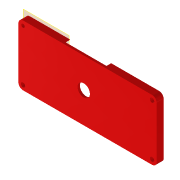
# Autodesk Inventor part: ESP32ParasiteMicroscope_top_v0
Saved by Autodesk Inventor 2022 (Build 260153000, 153)
## iProperties
Created: 2022-02-02
Part Number: ESP32ParasiteMicroscope_top_v0
Material: Generisch
Document SubType Name: Modeling
Designer: diederichbenedict
Density: 1 g/cm^3
Appearance: Rot
Author: diederichbenedict
Autodesk Inventor part; units mm, degrees
ref_plane "YZ Plane" through (0, 0, 0) normal (1, 0, 0) x (0, 1, 0)
ref_plane "XZ Plane" through (0, 0, 0) normal (0, 1, 0) x (-1, 0, 0)
ref_plane "XY Plane" through (0, 0, 0) normal (0, 0, 1) x (1, 0, 0)
ref_plane "Arbeitsebene1" through (0, 0, 0) normal (0, 0, 1) x (1, 0, 0)
sketch "Skizze1" plane through (0, 0, 0) normal (0, 0, 1) x (1, 0, 0)
  line L0 (-19.6031, 19.4874) -> (14.7153, 19.4874)
  line L1 (14.7153, -19.4874) -> (-19.6031, -19.4874)
  spline S0 degree 3 poles (15.9885, -12.7941) (15.1267, -14.0688) (14.121, -15.2558) (11.7288, -17.5435) (10.3143, -18.6047) (8.791, -19.4874) knots 0 0 0 0 0.461588 0.461588 0.987001 0.987001 0.987001 0.987001 projected
  line L2 (8.791, -19.4874) -> (41.5374, -19.4874) projected
  arc A0 (41.5374, -19.4874) -> (44.5374, -16.4874) centre (41.5374, -16.4874) ccw projected
  line L3 (44.5374, -16.4874) -> (44.5374, 16.4874) projected
  arc A1 (44.5374, 16.4874) -> (41.5374, 19.4874) centre (41.5374, 16.4874) ccw projected
  line L4 (41.5374, 19.4874) -> (7.7659, 19.4874) projected
  arc A2 (9.8338, 18.2553) -> (7.7659, 19.4874) centre (-2.4439, 0) ccw projected
  spline S1 degree 3 poles (9.8338, 18.2553) (12.0089, 16.8318) (13.9164, 15.0326) (17.1857, 10.6246) (18.4338, 7.9941) (19.8573, 2.3897) (20.014, -0.5318) (19.3704, -5.0763) (18.9435, -6.7188) (17.7261, -9.8803) (16.9385, -11.3888) (15.9885, -12.7941) knots 0.079909 0.079909 0.079909 0.079909 0.861026 0.861026 1.726159 1.726159 2.595399 2.595399 3.102699 3.102699 3.611409 3.611409 3.611409 3.611409 projected
  circle A3 centre (41.5374, 16.4874) radius 1.4 projected
  circle A4 centre (41.5374, -16.4874) radius 1.4 projected
  line L5 (7.9526, -13.3626) -> (-30.0474, -13.3626) projected
  spline S2 degree 3 poles (-21.9975, -11.0045) (-23.3957, -8.4471) (-24.2821, -5.6417) (-24.9256, 0.1377) (-24.6818, 3.0555) (-23.0907, 8.6196) (-21.7637, 11.2138) (-18.9405, 14.7925) (-17.7594, 15.9834) (-15.3624, 17.9058) (-14.189, 18.6758) (-12.951, 19.3288) knots 0 0 0 0 0.874402 0.874402 1.744697 1.744697 2.610882 2.610882 3.112603 3.112603 3.533005 3.533005 3.533005 3.533005 projected
  arc A5 (-12.6537, 19.4874) -> (-12.951, 19.3288) centre (-2.4439, 0) ccw projected
  line L6 (-12.6537, 19.4874) -> (-41.5374, 19.4874) projected
  arc A6 (-41.5374, 19.4874) -> (-44.5374, 16.4874) centre (-41.5374, 16.4874) ccw projected
  line L7 (-44.5374, 16.4874) -> (-44.5374, -16.4874) projected
  arc A7 (-44.5374, -16.4874) -> (-41.5374, -19.4874) centre (-41.5374, -16.4874) ccw projected
  line L8 (-41.5374, -19.4874) -> (-13.6864, -19.4874) projected
  spline S3 degree 3 poles (-13.6864, -19.4874) (-15.5675, -18.3989) (-17.2815, -17.0397) (-20.0302, -14.1081) (-21.1203, -12.6091) (-21.9975, -11.0045) knots 0.10415 0.10415 0.10415 0.10415 0.757219 0.757219 1.31027 1.31027 1.31027 1.31027 projected
  circle A8 centre (-41.5374, -16.4874) radius 1.4 projected
  circle A9 centre (-41.5374, 16.4874) radius 1.15 projected
  spline S4 degree 3 poles (-24.8057, 2.4903) (-24.4907, 5.3187) (-23.6418, 8.0626) (-20.9263, 13.1619) (-19.0572, 15.4543) (-14.5454, 19.1935) (-11.9459, 20.6045) (-6.3523, 22.3508) (-3.4117, 22.6693) (2.426, 22.1612) (5.2673, 21.3394) (10.4751, 18.653) (12.7917, 16.814) (16.5896, 12.3516) (18.0345, 9.7708) (19.8538, 4.2005) (20.2108, 1.2643) (19.7791, -4.5795) (18.9946, -7.4314) (16.3765, -12.6738) (14.568, -15.0143) (10.1556, -18.8702) (7.5939, -20.3489) (2.048, -22.2409) (-0.8833, -22.6362) (-6.7323, -22.281) (-9.5942, -21.5339) (-14.8704, -18.9846) (-17.2344, -17.2069) (-21.1477, -12.8453) (-22.6597, -10.3032) (-24.6241, -4.7825) (-25.0578, -1.8567) (-24.7791, 3.9965) (-24.0695, 6.8679) (-21.5895, 12.1771) (-19.8428, 14.564) (-15.5329, 18.5341) (-13.0107, 20.0793) (-7.5162, 22.1157) (-4.5963, 22.5876) (1.26, 22.3856) (4.1405, 21.7136) (9.4816, 19.3033) (11.8912, 17.588) (15.9174, 13.3303) (17.4954, 10.8286) (19.6036, 5.3612) (20.1136, 2.4477) (19.9882, -3.4108) (19.354, -6.2997) (17.0137, -11.672) (15.3301, -14.1038) (11.1255, -18.1853) (8.6447, -19.7959) (3.2053, -21.9755) (0.2987, -22.5236) (-5.5609, -22.4748) (-8.4579, -21.8784) (-13.8603, -19.6087) (-16.314, -17.957) (-20.4501, -13.8062) (-22.093, -11.3466) (-24.3436, -5.9362) (-24.9297, -3.0371) (-24.9576, 2.8227) (-24.3992, 5.7272) (-22.2003, 11.1588) (-20.5809, 13.6339) (-16.4845, 17.824) (-14.0467, 19.499) (-8.6662, 21.8201) (-5.7749, 22.4441) (0.0839, 22.5487) (2.9956, 22.0283) (8.4555, 19.9007) (10.9516, 18.3138) (15.1949, 14.2726) (16.9016, 11.8569) (19.2929, 6.5072) (19.9547, 3.6244) (20.1359, -2.2326) (19.6537, -5.1508) (17.5977, -10.6381) (16.0436, -13.1547) (12.0582, -17.4506) (9.665, -19.1887) (4.3471, -21.6499) (1.4732, -22.3493) (-4.3809, -22.6071) (-7.3052, -22.1631) (-12.8189, -20.1791) (-15.3556, -18.658) (-19.7032, -14.7292) (-21.4726, -12.359) (-24.0031, -7.0737) (-24.74, -4.2092) (-25.0745, 1.6411) (-24.6687, 4.5709) (-22.757, 10.1101) (-21.2693, 12.6665) (-17.3977, 17.0651) (-15.0508, 18.8653) (-9.7991, 21.4648) (-6.9445, 22.2391) (-1.0991, 22.6501) (1.8358, 22.2827) (7.3995, 20.4436) (9.9752, 18.9895) (14.4241, 15.1758) (16.2549, 12.8526) (18.9228, 7.6354) (19.7344, 4.7911) (20.2218, -1.0484) (19.8929, -3.9878) (18.1267, -9.5751) (16.7064, -12.1696) (12.9512, -16.668) (10.6523, -18.529) (6.0021, -20.9842) (3.7866, -21.7452) (-0.7988, -22.5603) (-3.1408, -22.6094) (-5.4486, -22.2985) knots 17.60465 17.60465 17.60465 17.60465 18.45888 18.45888 19.337874 19.337874 20.216868 20.216868 21.095862 21.095862 21.974857 21.974857 22.853851 22.853851 23.732845 23.732845 24.61184 24.61184 25.490834 25.490834 26.369828 26.369828 27.248822 27.248822 28.127817 28.127817 29.006811 29.006811 29.885805 29.885805 30.764799 30.764799 31.643794 31.643794 32.522788 32.522788 33.401782 33.401782 34.280777 34.280777 35.159771 35.159771 36.038765 36.038765 36.917759 36.917759 37.796754 37.796754 38.675748 38.675748 39.554742 39.554742 40.433736 40.433736 41.312731 41.312731 42.191725 42.191725 43.070719 43.070719 43.949713 43.949713 44.828708 44.828708 45.707702 45.707702 46.586696 46.586696 47.465691 47.465691 48.344685 48.344685 49.223679 49.223679 50.102673 50.102673 50.981668 50.981668 51.860662 51.860662 52.739656 52.739656 53.61865 53.61865 54.497645 54.497645 55.376639 55.376639 56.255633 56.255633 57.134628 57.134628 58.013622 58.013622 58.892616 58.892616 59.77161 59.77161 60.650605 60.650605 61.529599 61.529599 62.408593 62.408593 63.287587 63.287587 64.166582 64.166582 65.045576 65.045576 65.92457 65.92457 66.803564 66.803564 67.682559 67.682559 68.561553 68.561553 69.440547 69.440547 70.139143 70.139143 70.83774 70.83774 70.83774 70.83774 projected
  point P0 (0, 0)
  constraints: 4 end point, 1 horizontal, 1 parallel
extrude "Extrusion1" add sketch "Skizze1" along normal blind 4.5 contours A5 S2 S3 L5 S4 L0 | L0 A2 S1 S0 L1 S3 S2 A5 | L0 S4 L1 S0 S1 A2 | S4 L1 L8 A7 L7 A6 L6 L0 | L0 L4 A1 L3 A0 L2 L1 S4 | L5 S3 S4
sketch "Skizze2" plane through (0, 0, 0) normal (0, 0, -1) x (-1, 0, 0)
  spline S0 degree 3 poles (-8.6773, -19.4874) (-12.6741, -17.2065) (-15.9385, -13.664) (-17.8858, -9.4945) (-19.8263, -5.3394) (-20.4501, -0.581) (-19.646, 3.9338) (-18.841, 8.4547) (-16.6079, 12.7105) (-13.3453, 15.9419) (-11.953, 17.3208) (-10.3792, 18.5162) (-8.6773, 19.4874) knots 3.660178 3.660178 3.660178 3.660178 4.275468 4.275468 4.275468 4.888623 4.888623 4.888623 5.502599 5.502599 5.502599 5.7646 5.7646 5.7646 5.7646 projected
  spline S1 degree 3 poles (15.6702, -17.7105) (12.0344, -20.4258) (7.5456, -21.981) (3.0092, -22.097) (-1.5262, -22.2131) (-6.0878, -20.89) (-9.8573, -18.3651) (-13.6261, -15.8408) (-16.5853, -12.127) (-18.2044, -7.8897) (-19.8231, -3.6532) (-20.0946, 1.0867) (-18.9702, 5.4804) (-17.846, 9.8732) (-15.3316, 13.8993) (-11.8776, 16.8372) (-8.4243, 19.7746) (-4.0479, 21.6104) (0.4676, 22.0157) (4.9823, 22.421) (9.6148, 21.3945) (13.5357, 19.1199) (17.4559, 16.8457) (20.6463, 13.3346) (22.5357, 9.2152) (24.4248, 5.0964) (25.0045, 0.3887) (24.1711, -4.0654) (23.3017, -8.7119) (20.8952, -13.0574) (17.4179, -16.2597) (14.0494, -19.3619) (9.6951, -21.3773) (5.1502, -21.938) (0.6241, -22.4963) (-4.0691, -21.6096) (-8.0795, -19.4385) (-12.0876, -17.2687) (-15.3943, -13.8264) (-17.4015, -9.7344) (-19.4075, -5.6447) (-20.1058, -0.9257) (-19.3702, 3.5696) (-18.635, 8.0626) (-16.4709, 12.3107) (-13.2688, 15.547) (-10.0683, 18.7816) (-5.8461, 20.99) (-1.3638, 21.7738) (3.1163, 22.5573) (7.8349, 21.9139) (11.9417, 19.9597) (16.0466, 18.0064) (19.5207, 14.7528) (21.7387, 10.7848) (23.9556, 6.8185) (24.907, 2.1572) (24.4218, -2.3606) (23.9368, -6.8763) (22.0187, -11.2274) (19.0123, -14.6317) (16.0072, -18.0346) (11.9289, -20.4754) (7.5099, -21.5159) (3.0927, -22.556) (-1.6441, -22.1919) (-5.8505, -20.4891) (-10.0553, -18.7869) (-13.7102, -15.755) (-16.16, -11.9371) (-18.6088, -8.1206) (-19.8418, -3.5366) (-19.638, 0.9934) (-19.4343, 5.5218) (-17.7958, 9.975) (-15.0159, 13.5556) (-12.2369, 17.1349) (-8.3304, 19.8254) (-3.9954, 21.1455) (0.4165, 22.4891) (5.2511, 22.4051) (9.6138, 20.9091) (13.9256, 19.4306) (17.7557, 16.5809) (20.4109, 12.8758) (23.0632, 9.1748) (24.5305, 4.6381) (24.548, 0.0849) (24.5655, -4.4636) (23.136, -9.0069) (20.5173, -12.726) (17.9011, -16.4415) (14.1104, -19.3169) (9.8272, -20.8347) (5.5477, -22.3513) (0.7969, -22.5055) (-3.572, -21.2699) (-7.9373, -20.0352) (-11.9008, -17.4187) (-14.7514, -13.8896) (-17.6, -10.363) (-19.3241, -5.9418) (-19.6148, -1.4178) (-19.9144, 3.2433) (-18.6883, 7.9901) (-16.1689, 11.9231) (-13.7125, 15.7579) (-10.0405, 18.801) (-5.8164, 20.5028) (-1.6007, 22.2013) (3.1447, 22.5558) (7.5659, 21.5026) (11.9796, 20.4513) (16.0494, 18.0021) (19.0451, 14.5945) (22.1911, 11.016) (24.1323, 6.3965) (24.4869, 1.6449) (24.8252, -2.8882) (23.7216, -7.5182) (21.3749, -11.4113) (19.0355, -15.2922) (15.4721, -18.4228) (11.3223, -20.2429) (7.1708, -22.0637) (2.452, -22.5643) (-1.9891, -21.6552) (-2.6592, -21.518) (-3.3229, -21.3497) (-3.9774, -21.151) knots 24.602078 24.602078 24.602078 24.602078 25.217953 25.217953 25.217953 25.833709 25.833709 25.833709 26.449348 26.449348 26.449348 27.064873 27.064873 27.064873 27.680287 27.680287 27.680287 28.295593 28.295593 28.295593 28.910794 28.910794 28.910794 29.525892 29.525892 29.525892 30.140891 30.140891 30.140891 30.782458 30.782458 30.782458 31.403975 31.403975 31.403975 32.022909 32.022909 32.022909 32.641484 32.641484 32.641484 33.259714 33.259714 33.259714 33.87761 33.87761 33.87761 34.495185 34.495185 34.495185 35.11245 35.11245 35.11245 35.729418 35.729418 35.729418 36.346101 36.346101 36.346101 36.962511 36.962511 36.962511 37.578659 37.578659 37.578659 38.194557 38.194557 38.194557 38.810218 38.810218 38.810218 39.425653 39.425653 39.425653 40.040873 40.040873 40.040873 40.65589 40.65589 40.65589 41.281836 41.281836 41.281836 41.900486 41.900486 41.900486 42.518451 42.518451 42.518451 43.13578 43.13578 43.13578 43.752521 43.752521 43.752521 44.368723 44.368723 44.368723 44.984432 44.984432 44.984432 45.599696 45.599696 45.599696 46.233612 46.233612 46.233612 46.851689 46.851689 46.851689 47.468526 47.468526 47.468526 48.084314 48.084314 48.084314 48.730991 48.730991 48.730991 49.347941 49.347941 49.347941 49.962944 49.962944 49.962944 50.578193 50.578193 50.578193 50.671024 50.671024 50.671024 50.671024 projected
  circle A0 centre (2.4439, 0) radius 23.5
  point P0 (0, 0)
  dimension "d2" = 47
  constraints: 1 centre point, 1 coincident, 1 other
  measures "d2" diameter of A0
extrude "Extrusion2" cut sketch "Skizze2" against normal blind 3
sketch "Skizze3" plane through (0, 0, 4.5) normal (0, 0, 1) x (1, 0, 0)
  arc A0 (-15.5774, 19.4874) -> (-15.5774, -19.4874) centre (-2.4439, 0) ccw projected
  circle A1 centre (-2.4439, 0) radius 4
  point P0 (0, 0)
  dimension "d5" = 8
  constraints: 1 centre point, 1 coincident
  measures "d5" diameter of A1
extrude "Extrusion3" cut sketch "Skizze3" against normal blind 3
sketch "Skizze4" plane through (0, 0, 0) normal (0, 0, -1) x (-1, 0, 0)
  arc A0 (-10.6896, 19.4874) -> (-10.6896, -19.4874) centre (2.4439, 0) ccw projected
  line L0 (-41.5374, 19.4874) -> (-10.6896, 19.4874) projected
  arc A1 (-41.5374, 19.4874) -> (-44.5374, 16.4874) centre (-41.5374, 16.4874) ccw projected
  line L1 (-44.5374, -16.4874) -> (-44.5374, 16.4874) projected
  arc A2 (-44.5374, -16.4874) -> (-41.5374, -19.4874) centre (-41.5374, -16.4874) ccw projected
  line L2 (-10.6896, -19.4874) -> (-41.5374, -19.4874) projected
  circle A3 centre (-41.5374, -16.4874) radius 1.4 projected
  circle A4 centre (-41.5374, 16.4874) radius 1.4 projected
  arc A5 (15.5774, -19.4874) -> (15.5774, 19.4874) centre (2.4439, 0) ccw projected
  line L3 (41.5374, -19.4874) -> (15.5774, -19.4874) projected
  arc A6 (41.5374, -19.4874) -> (44.5374, -16.4874) centre (41.5374, -16.4874) ccw projected
  line L4 (44.5374, 16.4874) -> (44.5374, -16.4874) projected
  arc A7 (44.5374, 16.4874) -> (41.5374, 19.4874) centre (41.5374, 16.4874) ccw projected
  line L5 (15.5774, 19.4874) -> (41.5374, 19.4874) projected
  circle A8 centre (41.5374, 16.4874) radius 1.15 projected
  circle A9 centre (41.5374, -16.4874) radius 1.4 projected
  line L6 (32.5, -10) -> (-32.5, -10)
  line L7 (-32.5, -10) -> (-32.5, 10)
  line L8 (-32.5, 10) -> (32.5, 10)
  line L9 (32.5, 10) -> (32.5, -10)
  line L10 (32.5, -10) -> (-32.5, 10) construction
  line L11 (-32.5, -10) -> (32.5, 10) construction
  point P0 (0, 0)
  dimension "d8" = 65
  dimension "d9" = 20
  constraints: 12 end point, 2 midpoint, 2 parallel, 1 horizontal, 1 perpendicular
  measures "d8" distance of L7.end L8.end
  measures "d9" distance of L6.end L7.end
hole "Bohrung1" at (32.5, 10, 0) at (32.5, -10, 0) at (-32.5, 10, 0) at (-32.5, -10, 0) direction (0, 0, 1) diameter 8 depth 3.5
